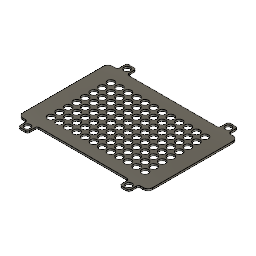
LEDSpacer_Gasket (Autodesk Fusion 360 design; units mm, degrees)
Autodesk Fusion 360 part; units mm, degrees
note: some values were not read from the file. Set by a fixed rule: which sketch regions a step uses.
sketch "Sketch1" plane through (0, 0, 0) normal (0, 0, 1) x (1, 0, 0)
  line L0 (-63.38, 47.37) -> (63.38, 47.37)
  line L1 (68.38, 42.37) -> (68.38, -42.37)
  line L2 (63.38, -47.37) -> (-63.38, -47.37)
  line L3 (-68.38, -42.37) -> (-68.38, 42.37)
  line L4 (-68.38, 47.37) -> (68.38, -47.37) construction
  line L5 (68.38, 47.37) -> (-68.38, -47.37) construction
  line L6 (-56.38, 57.37) -> (-50.38, 57.37)
  line L7 (-48.38, 55.37) -> (-48.38, 47.37)
  line L8 (-48.38, 47.37) -> (-58.38, 47.37)
  line L9 (-58.38, 47.37) -> (-58.38, 55.37)
  line L10 (50.38, 57.37) -> (56.38, 57.37)
  line L11 (58.38, 55.37) -> (58.38, 47.37)
  line L12 (58.38, 47.37) -> (48.38, 47.37)
  line L13 (48.38, 47.37) -> (48.38, 55.37)
  line L14 (48.38, -47.37) -> (58.38, -47.37)
  line L15 (58.38, -47.37) -> (58.38, -55.37)
  line L16 (56.38, -57.37) -> (50.38, -57.37)
  line L17 (48.38, -55.37) -> (48.38, -47.37)
  line L18 (-58.38, -47.37) -> (-48.38, -47.37)
  line L19 (-48.38, -47.37) -> (-48.38, -55.37)
  line L20 (-50.38, -57.37) -> (-56.38, -57.37)
  line L21 (-58.38, -55.37) -> (-58.38, -47.37)
  line L22 (-49.5, 31.5) -> (49.5, 31.5)
  line L23 (49.5, 31.5) -> (49.5, -31.5)
  line L24 (49.5, -31.5) -> (-49.5, -31.5)
  line L25 (-49.5, -31.5) -> (-49.5, 31.5)
  line L26 (-49.5, 31.5) -> (49.5, -31.5) construction
  line L27 (49.5, 31.5) -> (-49.5, -31.5) construction
  circle A0 centre (-49.5, -31.5) radius 3.575
  circle A1 centre (-40.5, -31.5) radius 3.575
  circle A2 centre (-31.5, -31.5) radius 3.575
  circle A3 centre (-22.5, -31.5) radius 3.575
  circle A4 centre (-13.5, -31.5) radius 3.575
  circle A5 centre (-4.5, -31.5) radius 3.575
  circle A6 centre (4.5, -31.5) radius 3.575
  circle A7 centre (13.5, -31.5) radius 3.575
  circle A8 centre (22.5, -31.5) radius 3.575
  circle A9 centre (31.5, -31.5) radius 3.575
  circle A10 centre (40.5, -31.5) radius 3.575
  circle A11 centre (49.5, -31.5) radius 3.575
  circle A12 centre (-49.5, -22.5) radius 3.575
  circle A13 centre (-40.5, -22.5) radius 3.575
  circle A14 centre (-31.5, -22.5) radius 3.575
  circle A15 centre (-22.5, -22.5) radius 3.575
  circle A16 centre (-13.5, -22.5) radius 3.575
  circle A17 centre (-4.5, -22.5) radius 3.575
  circle A18 centre (4.5, -22.5) radius 3.575
  circle A19 centre (13.5, -22.5) radius 3.575
  circle A20 centre (22.5, -22.5) radius 3.575
  circle A21 centre (31.5, -22.5) radius 3.575
  circle A22 centre (40.5, -22.5) radius 3.575
  circle A23 centre (49.5, -22.5) radius 3.575
  circle A24 centre (-49.5, -13.5) radius 3.575
  circle A25 centre (-40.5, -13.5) radius 3.575
  circle A26 centre (-31.5, -13.5) radius 3.575
  circle A27 centre (-22.5, -13.5) radius 3.575
  circle A28 centre (-13.5, -13.5) radius 3.575
  circle A29 centre (-4.5, -13.5) radius 3.575
  circle A30 centre (4.5, -13.5) radius 3.575
  circle A31 centre (13.5, -13.5) radius 3.575
  circle A32 centre (22.5, -13.5) radius 3.575
  circle A33 centre (31.5, -13.5) radius 3.575
  circle A34 centre (40.5, -13.5) radius 3.575
  circle A35 centre (49.5, -13.5) radius 3.575
  circle A36 centre (-49.5, -4.5) radius 3.575
  circle A37 centre (-40.5, -4.5) radius 3.575
  circle A38 centre (-31.5, -4.5) radius 3.575
  circle A39 centre (-22.5, -4.5) radius 3.575
  circle A40 centre (-13.5, -4.5) radius 3.575
  circle A41 centre (-4.5, -4.5) radius 3.575
  circle A42 centre (4.5, -4.5) radius 3.575
  circle A43 centre (13.5, -4.5) radius 3.575
  circle A44 centre (22.5, -4.5) radius 3.575
  circle A45 centre (31.5, -4.5) radius 3.575
  circle A46 centre (40.5, -4.5) radius 3.575
  circle A47 centre (49.5, -4.5) radius 3.575
  circle A48 centre (-49.5, 4.5) radius 3.575
  circle A49 centre (-40.5, 4.5) radius 3.575
  circle A50 centre (-31.5, 4.5) radius 3.575
  circle A51 centre (-22.5, 4.5) radius 3.575
  circle A52 centre (-13.5, 4.5) radius 3.575
  circle A53 centre (-4.5, 4.5) radius 3.575
  circle A54 centre (4.5, 4.5) radius 3.575
  circle A55 centre (13.5, 4.5) radius 3.575
  circle A56 centre (22.5, 4.5) radius 3.575
  circle A57 centre (31.5, 4.5) radius 3.575
  circle A58 centre (40.5, 4.5) radius 3.575
  circle A59 centre (49.5, 4.5) radius 3.575
  circle A60 centre (-49.5, 13.5) radius 3.575
  circle A61 centre (-40.5, 13.5) radius 3.575
  circle A62 centre (-31.5, 13.5) radius 3.575
  circle A63 centre (-22.5, 13.5) radius 3.575
  circle A64 centre (-13.5, 13.5) radius 3.575
  circle A65 centre (-4.5, 13.5) radius 3.575
  circle A66 centre (4.5, 13.5) radius 3.575
  circle A67 centre (13.5, 13.5) radius 3.575
  circle A68 centre (22.5, 13.5) radius 3.575
  circle A69 centre (31.5, 13.5) radius 3.575
  circle A70 centre (40.5, 13.5) radius 3.575
  circle A71 centre (49.5, 13.5) radius 3.575
  circle A72 centre (-49.5, 22.5) radius 3.575
  circle A73 centre (-40.5, 22.5) radius 3.575
  circle A74 centre (-31.5, 22.5) radius 3.575
  circle A75 centre (-22.5, 22.5) radius 3.575
  circle A76 centre (-13.5, 22.5) radius 3.575
  circle A77 centre (-4.5, 22.5) radius 3.575
  circle A78 centre (4.5, 22.5) radius 3.575
  circle A79 centre (13.5, 22.5) radius 3.575
  circle A80 centre (22.5, 22.5) radius 3.575
  circle A81 centre (31.5, 22.5) radius 3.575
  circle A82 centre (40.5, 22.5) radius 3.575
  circle A83 centre (49.5, 22.5) radius 3.575
  circle A84 centre (-49.5, 31.5) radius 3.575
  circle A85 centre (-40.5, 31.5) radius 3.575
  circle A86 centre (-31.5, 31.5) radius 3.575
  circle A87 centre (-22.5, 31.5) radius 3.575
  circle A88 centre (-13.5, 31.5) radius 3.575
  circle A89 centre (-4.5, 31.5) radius 3.575
  circle A90 centre (4.5, 31.5) radius 3.575
  circle A91 centre (13.5, 31.5) radius 3.575
  circle A92 centre (22.5, 31.5) radius 3.575
  circle A93 centre (31.5, 31.5) radius 3.575
  circle A94 centre (40.5, 31.5) radius 3.575
  circle A95 centre (49.5, 31.5) radius 3.575
  line L28 (-58.38, 57.37) -> (-53.38, 57.37)
  line L29 (-53.38, 57.37) -> (-53.38, 52.37)
  circle A96 centre (-53.38, 52.37) radius 3.25
  circle A97 centre (53.38, 52.37) radius 3.25
  circle A98 centre (-53.38, -52.37) radius 3.25
  circle A99 centre (53.38, -52.37) radius 3.25
  arc A100 (68.38, 42.37) -> (63.38, 47.37) centre (63.38, 42.37) ccw
  arc A101 (-63.38, 47.37) -> (-68.38, 42.37) centre (-63.38, 42.37) ccw
  arc A102 (-68.38, -42.37) -> (-63.38, -47.37) centre (-63.38, -42.37) ccw
  arc A103 (63.38, -47.37) -> (68.38, -42.37) centre (63.38, -42.37) ccw
  arc A104 (48.38, -55.37) -> (50.38, -57.37) centre (50.38, -55.37) ccw
  arc A105 (56.38, -57.37) -> (58.38, -55.37) centre (56.38, -55.37) ccw
  arc A106 (50.38, 57.37) -> (48.38, 55.37) centre (50.38, 55.37) ccw
  arc A107 (58.38, 55.37) -> (56.38, 57.37) centre (56.38, 55.37) ccw
  arc A108 (-56.38, 57.37) -> (-58.38, 55.37) centre (-56.38, 55.37) ccw
  arc A109 (-48.38, 55.37) -> (-50.38, 57.37) centre (-50.38, 55.37) ccw
  arc A110 (-58.38, -55.37) -> (-56.38, -57.37) centre (-56.38, -55.37) ccw
  arc A111 (-50.38, -57.37) -> (-48.38, -55.37) centre (-50.38, -55.37) ccw
  point P0 (-48.38, 57.37)
  point P1 (-57.3369, -42.2056)
  point P2 (-53.88, -84.89)
  point P3 (48.38, 57.37)
  point P4 (58.38, 57.37)
  dimension "d1" = 136.76
  dimension "d2" = 94.74
  dimension "d3" = 10
  dimension "d4" = 10
  dimension "d5" = 10
  dimension "d6" = 10
  dimension "d7" = 63
  dimension "d8" = 99
  dimension "d10" = 7.15
  dimension "d13" = 99
  dimension "d14" = 63
  dimension "d15" = 5
  dimension "d16" = 5
  dimension "d17" = 6.5
  dimension "d20" = 106.76
  dimension "d21" = -104.74
  dimension "d22" = 5
  dimension "d23" = 5
  dimension "d24" = 5
  dimension "d25" = 5
  dimension "d26" = 2
  dimension "d27" = 2
  dimension "d28" = 2
  dimension "d29" = 2
  dimension "d30" = 2
  constraint perpendicular L0 L1
  constraint parallel L0 L2
  constraint parallel L1 L3
  constraint horizontal L0
  constraint coincident L4 origin
  constraint coincident L5 origin
  constraint horizontal L6
  constraint vertical L7
  constraint horizontal L8
  constraint vertical L9
  constraint coincident L0 L7.end
  constraint horizontal L10
  constraint vertical L11
  constraint horizontal L12
  constraint vertical L13
  constraint horizontal L14
  constraint vertical L15
  constraint horizontal L16
  constraint vertical L17
  constraint horizontal L18
  constraint vertical L19
  constraint horizontal L20
  constraint vertical L21
  constraint perpendicular L22 L23
  constraint parallel L22 L24
  constraint parallel L23 L25
  constraint horizontal L22
  constraint coincident L26 origin
  constraint coincident L27 origin
  constraint perpendicular L9 L28
  constraint perpendicular L6 L29
  constraint coincident L29.end A96.centre
  constraint coincident L5.start L0
  constraint coincident L5.start L1
  constraint tangent L0 A100
  constraint tangent L1 A100
  constraint coincident L4.start L3
  constraint coincident L4.start L0
  constraint tangent L3 A101
  constraint tangent L0 A101
  constraint coincident L5.end L3
  constraint coincident L5.end L2
  constraint tangent L3 A102
  constraint tangent L2 A102
  constraint coincident L4.end L2
  constraint coincident L4.end L1
  constraint tangent L2 A103
  constraint tangent L1 A103
  constraint tangent L17 A104
  constraint tangent L16 A104
  constraint tangent L16 A105
  constraint tangent L15 A105
  constraint coincident P3 L13
  constraint coincident P3 L10
  constraint tangent L13 A106
  constraint tangent L10 A106
  constraint equal A105 A106
  constraint coincident P4 L11
  constraint coincident P4 L10
  constraint tangent L11 A107
  constraint tangent L10 A107
  constraint equal A105 A107
  constraint coincident L28.start L9
  constraint coincident L28.start L6
  constraint tangent L9 A108
  constraint tangent L6 A108
  constraint coincident P0 L7
  constraint coincident P0 L6
  constraint tangent L7 A109
  constraint tangent L6 A109
  constraint tangent L21 A110
  constraint tangent L20 A110
  constraint tangent L20 A111
  constraint tangent L19 A111
  constraint equal A110 A111
  measures "d1" distance of L1 L3
  measures "d2" distance of L4.start L5.end
  measures "d3" distance of L28.start P0
  measures "d4" distance of L28.start L8.end
  measures "d5" distance of P3 P4
  measures "d6" distance of P3 L12.end
  measures "d7" distance of L22.end L23.end
  measures "d8" distance of L23.end L24.end
  measures "d10" diameter of A0
  measures "d15" distance of L28.start L28.end
  measures "d16" distance of L28.end L29.end
  measures "d17" diameter of A96
  measures "d22" radius of A100
  measures "d23" radius of A101
  measures "d24" radius of A102
  measures "d25" radius of A103
  measures "d26" radius of A104
  measures "d27" radius of A105
  measures "d28" radius of A108
  measures "d29" radius of A109
  measures "d30" radius of A110
extrude "Extrude1" add sketch "Sketch1" along normal blind 2 contours L0 L1 L2 L3 L8 L12 L14 L18 A100 A101 A102 A103 | L0 L6 L7 L8 L9 L28 A108 A109 | L0 L10 L11 L12 L13 A106 A107 | L2 L18 L19 L20 L21 A110 A111 | L2 L14 L15 L16 L17 A104 A105 | L22 L23 L24 L25 A0 A1 A2 A3 A4 A5 A6 A7 A8 A9 A10 A11 A12 A23 A24 A35 A36 A47 A48 A59 A60 A71 A72 A83 A84 A85 A86 A87 A88 A89 A90 A91 A92 A93 A94 A95
fillet "Fillet1" radius 2 8 edges at (48.38, -47.37, 1) (-58.38, -47.37, 1) (58.38, -47.37, 1) (-48.38, -47.37, 1) (58.38, 47.37, 1) (-48.38, 47.37, 1) (-58.38, 47.37, 1) (48.38, 47.37, 1)
